Autodesk Fusion 360 part; units mm, degrees
(part 2 of 2)
sketch "スケッチ6" plane through (0, 0, 2) normal (0, 0, 1) x (-1, 0, 0)
  arc A0 (-43.4817, -98.8602) -> (-41.4947, -98.0676) centre (-42.8778, -97.4871) ccw
  arc A1 (41.4947, -98.0676) -> (-41.4947, -98.0676) centre (0, -115.48) ccw
  arc A2 (41.4947, -98.0676) -> (43.4817, -98.8602) centre (42.8778, -97.4871) ccw
  arc A3 (43.4817, -98.8602) -> (50.4167, -95.51) centre (0, 0) ccw
  arc A4 (50.4167, -95.51) -> (51.1376, -90.7356) centre (49.0163, -92.8569) ccw
  line L0 (51.1376, -90.7356) -> (40.8708, -80.4688)
  arc A5 (40.8708, -76.2261) -> (40.8708, -80.4688) centre (42.9921, -78.3474) ccw
  line L1 (40.8708, -76.2261) -> (76.2261, -40.8708)
  arc A6 (80.4688, -40.8708) -> (76.2261, -40.8708) centre (78.3474, -42.9921) ccw
  line L2 (80.4688, -40.8708) -> (90.7356, -51.1376)
  arc A7 (90.7356, -51.1376) -> (95.51, -50.4167) centre (92.8569, -49.0163) ccw
  arc A8 (95.51, -50.4167) -> (95.51, 50.4167) centre (0, 0) ccw
  arc A9 (95.51, 50.4167) -> (90.7356, 51.1376) centre (92.8569, 49.0163) ccw
  line L3 (90.7356, 51.1376) -> (80.4688, 40.8708)
  arc A10 (76.2261, 40.8708) -> (80.4688, 40.8708) centre (78.3474, 42.9921) ccw
  line L4 (76.2261, 40.8708) -> (40.8708, 76.2261)
  arc A11 (40.8708, 80.4688) -> (40.8708, 76.2261) centre (42.9921, 78.3474) ccw
  line L5 (40.8708, 80.4688) -> (51.1376, 90.7356)
  arc A12 (51.1376, 90.7356) -> (50.4167, 95.51) centre (49.0163, 92.8569) ccw
  arc A13 (50.4167, 95.51) -> (-50.4167, 95.51) centre (0, 0) ccw
  arc A14 (-50.4167, 95.51) -> (-51.1376, 90.7356) centre (-49.0163, 92.8569) ccw
  line L6 (-51.1376, 90.7356) -> (-40.8708, 80.4688)
  arc A15 (-40.8708, 76.2261) -> (-40.8708, 80.4688) centre (-42.9921, 78.3474) ccw
  line L7 (-40.8708, 76.2261) -> (-76.2261, 40.8708)
  arc A16 (-80.4688, 40.8708) -> (-76.2261, 40.8708) centre (-78.3474, 42.9921) ccw
  line L8 (-80.4688, 40.8708) -> (-90.7356, 51.1376)
  arc A17 (-90.7356, 51.1376) -> (-95.51, 50.4167) centre (-92.8569, 49.0163) ccw
  arc A18 (-95.51, 50.4167) -> (-95.51, -50.4167) centre (0, 0) ccw
  arc A19 (-95.51, -50.4167) -> (-90.7356, -51.1376) centre (-92.8569, -49.0163) ccw
  line L9 (-90.7356, -51.1376) -> (-80.4688, -40.8708)
  arc A20 (-76.2261, -40.8708) -> (-80.4688, -40.8708) centre (-78.3474, -42.9921) ccw
  line L10 (-76.2261, -40.8708) -> (-40.8708, -76.2261)
  arc A21 (-40.8708, -80.4688) -> (-40.8708, -76.2261) centre (-42.9921, -78.3474) ccw
  line L11 (-40.8708, -80.4688) -> (-51.1376, -90.7356)
  arc A22 (-51.1376, -90.7356) -> (-50.4167, -95.51) centre (-49.0163, -92.8569) ccw
  arc A23 (-50.4167, -95.51) -> (-43.4817, -98.8602) centre (0, 0) ccw
  arc A24 (-38.4462, 71.5797) -> (-36.9817, 75.1152) centre (-41.9817, 75.1152) ccw
  line L12 (-36.9817, 75.1152) -> (-36.9817, 81.5797)
  arc A25 (-36.9817, 81.5797) -> (-38.4462, 85.1152) centre (-41.9817, 81.5797) ccw
  line L13 (-38.4462, 85.1152) -> (-43.658, 90.3271)
  arc A26 (-43.0803, 93.5579) -> (-43.658, 90.3271) centre (-42.2438, 91.7413) ccw
  arc A27 (43.0803, 93.5579) -> (-43.0803, 93.5579) centre (0, 0) ccw
  arc A28 (43.658, 90.3271) -> (43.0803, 93.5579) centre (42.2438, 91.7413) ccw
  line L14 (43.658, 90.3271) -> (38.4462, 85.1152)
  arc A29 (38.4462, 85.1152) -> (36.9817, 81.5797) centre (41.9817, 81.5797) ccw
  line L15 (36.9817, 81.5797) -> (36.9817, 75.1152)
  arc A30 (36.9817, 75.1152) -> (38.4462, 71.5797) centre (41.9817, 75.1152) ccw
  line L16 (38.4462, 71.5797) -> (46.8812, 63.1446)
  arc A31 (46.8812, 58.902) -> (46.8812, 63.1446) centre (44.7599, 61.0233) ccw
  line L17 (46.8812, 58.902) -> (39.0462, 51.0671)
  arc A32 (35.1702, 49.6142) -> (39.0462, 51.0671) centre (35.5107, 54.6026) ccw
  arc A33 (35.1702, 49.6142) -> (32.5058, 46.9498) centre (35, 47.12) ccw
  arc A34 (31.0529, 43.0738) -> (32.5058, 46.9498) centre (27.5174, 46.6093) ccw
  line L18 (31.0529, 43.0738) -> (11.7378, 23.7586)
  arc A35 (11.7378, 23.7586) -> (-9.9511, 24.5606) centre (0, 0) ccw
  arc A36 (-13.199, 25.2198) -> (-9.9511, 24.5606) centre (-11.0776, 27.3411) ccw
  line L19 (-13.199, 25.2198) -> (-31.0529, 43.0738)
  arc A37 (-32.5058, 46.9498) -> (-31.0529, 43.0738) centre (-27.5174, 46.6093) ccw
  arc A38 (-32.5058, 46.9498) -> (-35.1702, 49.6142) centre (-35, 47.12) ccw
  arc A39 (-39.0462, 51.0671) -> (-35.1702, 49.6142) centre (-35.5107, 54.6026) ccw
  line L20 (-39.0462, 51.0671) -> (-46.8812, 58.902)
  arc A40 (-46.8812, 63.1446) -> (-46.8812, 58.902) centre (-44.7599, 61.0233) ccw
  line L21 (-46.8812, 63.1446) -> (-38.4462, 71.5797)
  arc A41 (-72.6906, -37.3352) -> (-84.0043, -37.3352) centre (-78.3474, -42.9921) ccw
  line L22 (-84.0043, -37.3352) -> (-90.3271, -43.658)
  arc A42 (-93.5579, -43.0803) -> (-90.3271, -43.658) centre (-91.7413, -42.2438) ccw
  arc A43 (-93.5579, 43.0803) -> (-93.5579, -43.0803) centre (0, 0) ccw
  arc A44 (-90.3271, 43.658) -> (-93.5579, 43.0803) centre (-91.7413, 42.2438) ccw
  line L23 (-90.3271, 43.658) -> (-84.0043, 37.3352)
  arc A45 (-84.0043, 37.3352) -> (-72.6906, 37.3352) centre (-78.3474, 42.9921) ccw
  line L24 (-72.6906, 37.3352) -> (-63.1446, 46.8812)
  arc A46 (-58.902, 46.8812) -> (-63.1446, 46.8812) centre (-61.0233, 44.7599) ccw
  line L25 (-58.902, 46.8812) -> (-42.5942, 30.5734)
  arc A47 (-42.1845, 26.8416) -> (-42.5942, 30.5734) centre (-44.7155, 28.4521) ccw
  arc A48 (-42.1845, 26.8416) -> (-42.1845, -26.8416) centre (0, 0) ccw
  arc A49 (-42.5942, -30.5734) -> (-42.1845, -26.8416) centre (-44.7155, -28.4521) ccw
  line L26 (-42.5942, -30.5734) -> (-58.902, -46.8812)
  arc A50 (-63.1446, -46.8812) -> (-58.902, -46.8812) centre (-61.0233, -44.7599) ccw
  line L27 (-63.1446, -46.8812) -> (-72.6906, -37.3352)
  arc A51 (72.6906, 37.3352) -> (84.0043, 37.3352) centre (78.3474, 42.9921) ccw
  line L28 (84.0043, 37.3352) -> (90.3271, 43.658)
  arc A52 (93.5579, 43.0803) -> (90.3271, 43.658) centre (91.7413, 42.2438) ccw
  arc A53 (93.5579, -43.0803) -> (93.5579, 43.0803) centre (0, 0) ccw
  arc A54 (90.3271, -43.658) -> (93.5579, -43.0803) centre (91.7413, -42.2438) ccw
  line L29 (90.3271, -43.658) -> (84.0043, -37.3352)
  arc A55 (84.0043, -37.3352) -> (72.6906, -37.3352) centre (78.3474, -42.9921) ccw
  line L30 (72.6906, -37.3352) -> (63.1446, -46.8812)
  arc A56 (58.902, -46.8812) -> (63.1446, -46.8812) centre (61.0233, -44.7599) ccw
  line L31 (58.902, -46.8812) -> (42.5942, -30.5734)
  arc A57 (42.1845, -26.8416) -> (42.5942, -30.5734) centre (44.7155, -28.4521) ccw
  arc A58 (42.1845, -26.8416) -> (42.1845, 26.8416) centre (0, 0) ccw
  arc A59 (42.5942, 30.5734) -> (42.1845, 26.8416) centre (44.7155, 28.4521) ccw
  line L32 (42.5942, 30.5734) -> (58.902, 46.8812)
  arc A60 (63.1446, 46.8812) -> (58.902, 46.8812) centre (61.0233, 44.7599) ccw
  line L33 (63.1446, 46.8812) -> (72.6906, 37.3352)
  line L34 (-22.2194, 14.4412) -> (-56.7807, 49.0025)
  arc A61 (-56.7807, 53.2451) -> (-56.7807, 49.0025) centre (-54.6594, 51.1238) ccw
  line L35 (-56.7807, 53.2451) -> (-53.2451, 56.7807)
  arc A62 (-49.0025, 56.7807) -> (-53.2451, 56.7807) centre (-51.1238, 54.6594) ccw
  line L36 (-49.0025, 56.7807) -> (-14.4412, 22.2194)
  arc A63 (-14.4412, 22.2194) -> (-22.2194, 14.4412) centre (0, 0) ccw
  circle A64 centre (-92.7295, 48.1818) radius 1.65
  circle A65 centre (-92.7295, -48.1818) radius 1.65
  line L37 (-34.5739, 22.5531) -> (-26.135, 14.1142)
  arc A66 (-24.9609, 8.8995) -> (-26.135, 14.1142) centre (-29.6706, 10.5787) ccw
  arc A67 (-24.9609, 8.8995) -> (-24.9609, -8.8995) centre (0, 0) ccw
  arc A68 (-26.135, -14.1142) -> (-24.9609, -8.8995) centre (-29.6706, -10.5787) ccw
  line L38 (-26.135, -14.1142) -> (-34.5739, -22.5531)
  arc A69 (-39.3163, -21.8912) -> (-34.5739, -22.5531) centre (-36.6953, -20.4318) ccw
  arc A70 (-39.3163, 21.8912) -> (-39.3163, -21.8912) centre (0, 0) ccw
  arc A71 (-34.5739, 22.5531) -> (-39.3163, 21.8912) centre (-36.6953, 20.4318) ccw
  line L39 (-56.7807, -49.0025) -> (-22.2194, -14.4412)
  arc A72 (-22.2194, -14.4412) -> (-14.4412, -22.2194) centre (0, 0) ccw
  line L40 (-14.4412, -22.2194) -> (-31.1442, -38.9224)
  arc A73 (-34.8932, -40.3823) -> (-31.1442, -38.9224) centre (-34.6797, -35.3868) ccw
  arc A74 (-34.8932, -40.3823) -> (-37.4977, -42.9868) centre (-35, -42.88) ccw
  arc A75 (-38.9576, -46.7358) -> (-37.4977, -42.9868) centre (-42.4932, -43.2003) ccw
  line L41 (-38.9576, -46.7358) -> (-49.0025, -56.7807)
  arc A76 (-53.2451, -56.7807) -> (-49.0025, -56.7807) centre (-51.1238, -54.6594) ccw
  line L42 (-53.2451, -56.7807) -> (-56.7807, -53.2451)
  arc A77 (-56.7807, -49.0025) -> (-56.7807, -53.2451) centre (-54.6594, -51.1238) ccw
  circle A78 centre (-48.1818, -92.7295) radius 1.65
  circle A79 centre (48.1818, -92.7295) radius 1.65
  arc A80 (23.7586, -11.7378) -> (23.7586, 11.7378) centre (0, 0) ccw
  line L43 (23.7586, 11.7378) -> (34.5739, 22.5531)
  arc A81 (39.3163, 21.8912) -> (34.5739, 22.5531) centre (36.6953, 20.4318) ccw
  arc A82 (39.3163, -21.8912) -> (39.3163, 21.8912) centre (0, 0) ccw
  arc A83 (34.5739, -22.5531) -> (39.3163, -21.8912) centre (36.6953, -20.4318) ccw
  line L44 (34.5739, -22.5531) -> (23.7586, -11.7378)
  circle A84 centre (48.1818, 92.7295) radius 1.65
  circle A85 centre (35, 47.12) radius 1.65
  circle A86 centre (-35, 47.12) radius 1.65
  circle A87 centre (45.7881, -12.6183) radius 1.65
  circle A88 centre (35, -42.88) radius 1.65
  line L45 (22.2194, -14.4412) -> (56.7807, -49.0025)
  arc A89 (56.7807, -53.2451) -> (56.7807, -49.0025) centre (54.6594, -51.1238) ccw
  line L46 (56.7807, -53.2451) -> (53.2451, -56.7807)
  arc A90 (49.0025, -56.7807) -> (53.2451, -56.7807) centre (51.1238, -54.6594) ccw
  line L47 (49.0025, -56.7807) -> (38.9576, -46.7358)
  arc A91 (37.4977, -42.9868) -> (38.9576, -46.7358) centre (42.4932, -43.2003) ccw
  arc A92 (37.4977, -42.9868) -> (34.8932, -40.3823) centre (35, -42.88) ccw
  arc A93 (31.1442, -38.9224) -> (34.8932, -40.3823) centre (34.6797, -35.3868) ccw
  line L48 (31.1442, -38.9224) -> (14.4412, -22.2194)
  arc A94 (14.4412, -22.2194) -> (22.2194, -14.4412) centre (0, 0) ccw
  circle A95 centre (92.7295, -48.1818) radius 1.65
  circle A96 centre (92.7295, 48.1818) radius 1.65
  line L49 (53.2451, 56.7807) -> (56.7807, 53.2451)
  arc A97 (56.7807, 49.0025) -> (56.7807, 53.2451) centre (54.6594, 51.1238) ccw
  line L50 (56.7807, 49.0025) -> (22.2194, 14.4412)
  arc A98 (22.2194, 14.4412) -> (14.4412, 22.2194) centre (0, 0) ccw
  line L51 (14.4412, 22.2194) -> (49.0025, 56.7807)
  arc A99 (53.2451, 56.7807) -> (49.0025, 56.7807) centre (51.1238, 54.6594) ccw
  line L52 (9, -66.2967) -> (9, -24.9249)
  line L53 (11.7378, -23.7586) -> (46.8812, -58.902)
  arc A100 (46.8812, -63.1446) -> (46.8812, -58.902) centre (44.7599, -61.0233) ccw
  line L54 (46.8812, -63.1446) -> (34.4346, -75.5912)
  arc A101 (30.4842, -75.8478) -> (34.4346, -75.5912) centre (32.3133, -73.4699) ccw
  arc A102 (30.4842, -75.8478) -> (9, -66.2967) centre (0, -115.48) ccw
  arc A103 (6, -65.8413) -> (-6, -65.8413) centre (0, -115.48) ccw
  line L55 (-6, -65.8413) -> (-6, -25.8118)
  arc A104 (-6, -25.8118) -> (6, -25.8118) centre (0, 0) ccw
  line L56 (6, -25.8118) -> (6, -65.8413)
  circle A105 centre (-45.7881, -12.6183) radius 1.65
  line L57 (-46.8812, -58.902) -> (-11.7378, -23.7586)
  line L58 (-9, -24.9249) -> (-9, -66.2967)
  arc A106 (-9, -66.2967) -> (-30.4842, -75.8478) centre (0, -115.48) ccw
  arc A107 (-34.4346, -75.5912) -> (-30.4842, -75.8478) centre (-32.3133, -73.4699) ccw
  line L59 (-34.4346, -75.5912) -> (-46.8812, -63.1446)
  arc A108 (-46.8812, -58.902) -> (-46.8812, -63.1446) centre (-44.7599, -61.0233) ccw
  circle A109 centre (-35, -42.88) radius 1.65
  circle A110 centre (0, 0) radius 23.5
  circle A111 centre (-48.1818, 92.7295) radius 1.65
  line L60 (43.2721, 31.2513) -> (33.8603, 21.8395)
  circle A112 centre (0, 0) radius 50
  circle A113 centre (0, 0) radius 45
  line L61 (40.8511, 28.8303) -> (43.8511, 28.8303)
  circle A114 centre (43.8511, 28.8303) radius 2.5
  circle A115 centre (43.8511, 28.8303) radius 1.65
  line L62 (0, -2.5) -> (0, -20)
  circle A116 centre (-43.8511, 28.8303) radius 2.5
  circle A117 centre (-43.8511, 28.8303) radius 1.65
  arc A118 (9, -24.9249) -> (11.7378, -23.7586) centre (0, 0) ccw
  arc A119 (-11.7378, -23.7586) -> (-9, -24.9249) centre (0, 0) ccw
  dimension "d249" = 3
  dimension "d250" = 5
  dimension "d251" = 3.3
  constraint coincident L32 L60.start
  constraint coincident L43 L60.end
  constraint concentric A3 A112
  constraint coincident A3.centre A8.centre
  constraint coincident A112 L61.start
  constraint coincident L60 L61.start
  constraint horizontal L61
  constraint coincident L61.end A114.centre
  constraint concentric A114 A115
  constraint symmetric A114 L62 A116
  constraint symmetric A115 L62 A117
  measures "d249" distance of L61.start L61.end
  measures "d250" diameter of A114
  measures "d251" diameter of A115
extrude "押し出し9" add sketch "スケッチ6" against normal blind 2 contours L25 A47 A116 | A59 L32 L60 A114
fillet "フィレット34" radius 3 2 edges at (-23.7586, 11.7378, 1) (-23.7586, -11.7378, 1)
fillet "フィレット35" radius 4 4 edges at (-42.0273, -27.1204, 1) (-43.2865, -31.2657, 1) (43.2865, -31.2657, 1) (42.0273, -27.1204, 1)
sketch "スケッチ7" plane through (0, 0, 2) normal (0, 0, 1) x (-1, 0, 0)
  circle A0 centre (-43.8511, 28.8303) radius 1.65
  circle A1 centre (43.8511, 28.8303) radius 1.65
  arc A2 (-43.4817, -98.8602) -> (-41.4947, -98.0676) centre (-42.8778, -97.4871) ccw
  arc A3 (41.4947, -98.0676) -> (-41.4947, -98.0676) centre (0, -115.48) ccw
  arc A4 (41.4947, -98.0676) -> (43.4817, -98.8602) centre (42.8778, -97.4871) ccw
  arc A5 (43.4817, -98.8602) -> (50.4167, -95.51) centre (0, 0) ccw
  arc A6 (50.4167, -95.51) -> (51.1376, -90.7356) centre (49.0163, -92.8569) ccw
  line L0 (51.1376, -90.7356) -> (40.8708, -80.4688)
  arc A7 (40.8708, -76.2261) -> (40.8708, -80.4688) centre (42.9921, -78.3474) ccw
  line L1 (40.8708, -76.2261) -> (76.2261, -40.8708)
  arc A8 (80.4688, -40.8708) -> (76.2261, -40.8708) centre (78.3474, -42.9921) ccw
  line L2 (80.4688, -40.8708) -> (90.7356, -51.1376)
  arc A9 (90.7356, -51.1376) -> (95.51, -50.4167) centre (92.8569, -49.0163) ccw
  arc A10 (95.51, -50.4167) -> (95.51, 50.4167) centre (0, 0) ccw
  arc A11 (95.51, 50.4167) -> (90.7356, 51.1376) centre (92.8569, 49.0163) ccw
  line L3 (90.7356, 51.1376) -> (80.4688, 40.8708)
  arc A12 (76.2261, 40.8708) -> (80.4688, 40.8708) centre (78.3474, 42.9921) ccw
  line L4 (76.2261, 40.8708) -> (40.8708, 76.2261)
  arc A13 (40.8708, 80.4688) -> (40.8708, 76.2261) centre (42.9921, 78.3474) ccw
  line L5 (40.8708, 80.4688) -> (51.1376, 90.7356)
  arc A14 (51.1376, 90.7356) -> (50.4167, 95.51) centre (49.0163, 92.8569) ccw
  arc A15 (50.4167, 95.51) -> (-50.4167, 95.51) centre (0, 0) ccw
  arc A16 (-50.4167, 95.51) -> (-51.1376, 90.7356) centre (-49.0163, 92.8569) ccw
  line L6 (-51.1376, 90.7356) -> (-40.8708, 80.4688)
  arc A17 (-40.8708, 76.2261) -> (-40.8708, 80.4688) centre (-42.9921, 78.3474) ccw
  line L7 (-40.8708, 76.2261) -> (-76.2261, 40.8708)
  arc A18 (-80.4688, 40.8708) -> (-76.2261, 40.8708) centre (-78.3474, 42.9921) ccw
  line L8 (-80.4688, 40.8708) -> (-90.7356, 51.1376)
  arc A19 (-90.7356, 51.1376) -> (-95.51, 50.4167) centre (-92.8569, 49.0163) ccw
  arc A20 (-95.51, 50.4167) -> (-95.51, -50.4167) centre (0, 0) ccw
  arc A21 (-95.51, -50.4167) -> (-90.7356, -51.1376) centre (-92.8569, -49.0163) ccw
  line L9 (-90.7356, -51.1376) -> (-80.4688, -40.8708)
  arc A22 (-76.2261, -40.8708) -> (-80.4688, -40.8708) centre (-78.3474, -42.9921) ccw
  line L10 (-76.2261, -40.8708) -> (-40.8708, -76.2261)
  arc A23 (-40.8708, -80.4688) -> (-40.8708, -76.2261) centre (-42.9921, -78.3474) ccw
  line L11 (-40.8708, -80.4688) -> (-51.1376, -90.7356)
  arc A24 (-51.1376, -90.7356) -> (-50.4167, -95.51) centre (-49.0163, -92.8569) ccw
  arc A25 (-50.4167, -95.51) -> (-43.4817, -98.8602) centre (0, 0) ccw
  arc A26 (-38.4462, 71.5797) -> (-36.9817, 75.1152) centre (-41.9817, 75.1152) ccw
  line L12 (-36.9817, 75.1152) -> (-36.9817, 81.5797)
  arc A27 (-36.9817, 81.5797) -> (-38.4462, 85.1152) centre (-41.9817, 81.5797) ccw
  line L13 (-38.4462, 85.1152) -> (-43.658, 90.3271)
  arc A28 (-43.0803, 93.5579) -> (-43.658, 90.3271) centre (-42.2438, 91.7413) ccw
  arc A29 (43.0803, 93.5579) -> (-43.0803, 93.5579) centre (0, 0) ccw
  arc A30 (43.658, 90.3271) -> (43.0803, 93.5579) centre (42.2438, 91.7413) ccw
  line L14 (43.658, 90.3271) -> (38.4462, 85.1152)
  arc A31 (38.4462, 85.1152) -> (36.9817, 81.5797) centre (41.9817, 81.5797) ccw
  line L15 (36.9817, 81.5797) -> (36.9817, 75.1152)
  arc A32 (36.9817, 75.1152) -> (38.4462, 71.5797) centre (41.9817, 75.1152) ccw
  line L16 (38.4462, 71.5797) -> (46.8812, 63.1446)
  arc A33 (46.8812, 58.902) -> (46.8812, 63.1446) centre (44.7599, 61.0233) ccw
  line L17 (46.8812, 58.902) -> (39.0462, 51.0671)
  arc A34 (35.1702, 49.6142) -> (39.0462, 51.0671) centre (35.5107, 54.6026) ccw
  arc A35 (35.1702, 49.6142) -> (32.5058, 46.9498) centre (35, 47.12) ccw
  arc A36 (31.0529, 43.0738) -> (32.5058, 46.9498) centre (27.5174, 46.6093) ccw
  line L18 (31.0529, 43.0738) -> (11.7378, 23.7586)
  arc A37 (11.7378, 23.7586) -> (-9.9511, 24.5606) centre (0, 0) ccw
  arc A38 (-13.199, 25.2198) -> (-9.9511, 24.5606) centre (-11.0776, 27.3411) ccw
  line L19 (-13.199, 25.2198) -> (-31.0529, 43.0738)
  arc A39 (-32.5058, 46.9498) -> (-31.0529, 43.0738) centre (-27.5174, 46.6093) ccw
  arc A40 (-32.5058, 46.9498) -> (-35.1702, 49.6142) centre (-35, 47.12) ccw
  arc A41 (-39.0462, 51.0671) -> (-35.1702, 49.6142) centre (-35.5107, 54.6026) ccw
  line L20 (-39.0462, 51.0671) -> (-46.8812, 58.902)
  arc A42 (-46.8812, 63.1446) -> (-46.8812, 58.902) centre (-44.7599, 61.0233) ccw
  line L21 (-46.8812, 63.1446) -> (-38.4462, 71.5797)
  arc A43 (-72.6906, -37.3352) -> (-84.0043, -37.3352) centre (-78.3474, -42.9921) ccw
  line L22 (-84.0043, -37.3352) -> (-90.3271, -43.658)
  arc A44 (-93.5579, -43.0803) -> (-90.3271, -43.658) centre (-91.7413, -42.2438) ccw
  arc A45 (-93.5579, 43.0803) -> (-93.5579, -43.0803) centre (0, 0) ccw
  arc A46 (-90.3271, 43.658) -> (-93.5579, 43.0803) centre (-91.7413, 42.2438) ccw
  line L23 (-90.3271, 43.658) -> (-84.0043, 37.3352)
  arc A47 (-84.0043, 37.3352) -> (-72.6906, 37.3352) centre (-78.3474, 42.9921) ccw
  line L24 (-72.6906, 37.3352) -> (-63.1446, 46.8812)
  arc A48 (-58.902, 46.8812) -> (-63.1446, 46.8812) centre (-61.0233, 44.7599) ccw
  line L25 (-58.902, 46.8812) -> (-46.7511, 34.7303)
  arc A49 (-46.0544, 30.0117) -> (-46.7511, 34.7303) centre (-49.5796, 31.9019) ccw
  arc A50 (-46.0544, 30.0117) -> (-45.5696, 27.0146) centre (-43.8511, 28.8303) ccw
  arc A51 (-44.7399, 22.3235) -> (-45.5696, 27.0146) centre (-48.3191, 24.1094) ccw
  arc A52 (-44.7399, 22.3235) -> (-42.1845, -26.8416) centre (0, 0) ccw
  arc A53 (-42.5942, -30.5734) -> (-42.1845, -26.8416) centre (-44.7155, -28.4521) ccw
  line L26 (-42.5942, -30.5734) -> (-58.902, -46.8812)
  arc A54 (-63.1446, -46.8812) -> (-58.902, -46.8812) centre (-61.0233, -44.7599) ccw
  line L27 (-63.1446, -46.8812) -> (-72.6906, -37.3352)
  arc A55 (72.6906, 37.3352) -> (84.0043, 37.3352) centre (78.3474, 42.9921) ccw
  line L28 (84.0043, 37.3352) -> (90.3271, 43.658)
  arc A56 (93.5579, 43.0803) -> (90.3271, 43.658) centre (91.7413, 42.2438) ccw
  arc A57 (93.5579, -43.0803) -> (93.5579, 43.0803) centre (0, 0) ccw
  arc A58 (90.3271, -43.658) -> (93.5579, -43.0803) centre (91.7413, -42.2438) ccw
  line L29 (90.3271, -43.658) -> (84.0043, -37.3352)
  arc A59 (84.0043, -37.3352) -> (72.6906, -37.3352) centre (78.3474, -42.9921) ccw
  line L30 (72.6906, -37.3352) -> (63.1446, -46.8812)
  arc A60 (58.902, -46.8812) -> (63.1446, -46.8812) centre (61.0233, -44.7599) ccw
  line L31 (58.902, -46.8812) -> (42.5942, -30.5734)
  arc A61 (42.1845, -26.8416) -> (42.5942, -30.5734) centre (44.7155, -28.4521) ccw
  arc A62 (42.1845, -26.8416) -> (44.7399, 22.3235) centre (0, 0) ccw
  arc A63 (45.5696, 27.0146) -> (44.7399, 22.3235) centre (48.3191, 24.1094) ccw
  arc A64 (45.5696, 27.0146) -> (46.0544, 30.0117) centre (43.8511, 28.8303) ccw
  arc A65 (46.7511, 34.7303) -> (46.0544, 30.0117) centre (49.5796, 31.9019) ccw
  line L32 (46.7511, 34.7303) -> (58.902, 46.8812)
  arc A66 (63.1446, 46.8812) -> (58.902, 46.8812) centre (61.0233, 44.7599) ccw
  line L33 (63.1446, 46.8812) -> (72.6906, 37.3352)
  line L34 (-22.2194, 14.4412) -> (-56.7807, 49.0025)
  arc A67 (-56.7807, 53.2451) -> (-56.7807, 49.0025) centre (-54.6594, 51.1238) ccw
  line L35 (-56.7807, 53.2451) -> (-53.2451, 56.7807)
  arc A68 (-49.0025, 56.7807) -> (-53.2451, 56.7807) centre (-51.1238, 54.6594) ccw
  line L36 (-49.0025, 56.7807) -> (-14.4412, 22.2194)
  arc A69 (-14.4412, 22.2194) -> (-22.2194, 14.4412) centre (0, 0) ccw
  circle A70 centre (-92.7295, 48.1818) radius 1.65
  circle A71 centre (-92.7295, -48.1818) radius 1.65
  line L37 (-34.5739, 22.5531) -> (-26.135, 14.1142)
  arc A72 (-24.9609, 8.8995) -> (-26.135, 14.1142) centre (-29.6706, 10.5787) ccw
  arc A73 (-24.9609, 8.8995) -> (-24.9609, -8.8995) centre (0, 0) ccw
  arc A74 (-26.135, -14.1142) -> (-24.9609, -8.8995) centre (-29.6706, -10.5787) ccw
  line L38 (-26.135, -14.1142) -> (-34.5739, -22.5531)
  arc A75 (-39.3163, -21.8912) -> (-34.5739, -22.5531) centre (-36.6953, -20.4318) ccw
  arc A76 (-39.3163, 21.8912) -> (-39.3163, -21.8912) centre (0, 0) ccw
  arc A77 (-34.5739, 22.5531) -> (-39.3163, 21.8912) centre (-36.6953, 20.4318) ccw
  line L39 (-56.7807, -49.0025) -> (-22.2194, -14.4412)
  arc A78 (-22.2194, -14.4412) -> (-14.4412, -22.2194) centre (0, 0) ccw
  line L40 (-14.4412, -22.2194) -> (-31.1442, -38.9224)
  arc A79 (-34.8932, -40.3823) -> (-31.1442, -38.9224) centre (-34.6797, -35.3868) ccw
  arc A80 (-34.8932, -40.3823) -> (-37.4977, -42.9868) centre (-35, -42.88) ccw
  arc A81 (-38.9576, -46.7358) -> (-37.4977, -42.9868) centre (-42.4932, -43.2003) ccw
  line L41 (-38.9576, -46.7358) -> (-49.0025, -56.7807)
  arc A82 (-53.2451, -56.7807) -> (-49.0025, -56.7807) centre (-51.1238, -54.6594) ccw
  line L42 (-53.2451, -56.7807) -> (-56.7807, -53.2451)
  arc A83 (-56.7807, -49.0025) -> (-56.7807, -53.2451) centre (-54.6594, -51.1238) ccw
  circle A84 centre (-48.1818, -92.7295) radius 1.65
  circle A85 centre (48.1818, -92.7295) radius 1.65
  arc A86 (24.5606, -9.9511) -> (24.5606, 9.9511) centre (0, 0) ccw
  arc A87 (25.2198, 13.199) -> (24.5606, 9.9511) centre (27.3411, 11.0776) ccw
  line L43 (25.2198, 13.199) -> (34.5739, 22.5531)
  arc A88 (39.3163, 21.8912) -> (34.5739, 22.5531) centre (36.6953, 20.4318) ccw
  arc A89 (39.3163, -21.8912) -> (39.3163, 21.8912) centre (0, 0) ccw
  arc A90 (34.5739, -22.5531) -> (39.3163, -21.8912) centre (36.6953, -20.4318) ccw
  line L44 (34.5739, -22.5531) -> (25.2198, -13.199)
  arc A91 (24.5606, -9.9511) -> (25.2198, -13.199) centre (27.3411, -11.0776) ccw
  circle A92 centre (48.1818, 92.7295) radius 1.65
  circle A93 centre (35, 47.12) radius 1.65
  circle A94 centre (-35, 47.12) radius 1.65
  circle A95 centre (45.7881, -12.6183) radius 1.65
  circle A96 centre (35, -42.88) radius 1.65
  line L45 (22.2194, -14.4412) -> (56.7807, -49.0025)
  arc A97 (56.7807, -53.2451) -> (56.7807, -49.0025) centre (54.6594, -51.1238) ccw
  line L46 (56.7807, -53.2451) -> (53.2451, -56.7807)
  arc A98 (49.0025, -56.7807) -> (53.2451, -56.7807) centre (51.1238, -54.6594) ccw
  line L47 (49.0025, -56.7807) -> (38.9576, -46.7358)
  arc A99 (37.4977, -42.9868) -> (38.9576, -46.7358) centre (42.4932, -43.2003) ccw
  arc A100 (37.4977, -42.9868) -> (34.8932, -40.3823) centre (35, -42.88) ccw
  arc A101 (31.1442, -38.9224) -> (34.8932, -40.3823) centre (34.6797, -35.3868) ccw
  line L48 (31.1442, -38.9224) -> (14.4412, -22.2194)
  arc A102 (14.4412, -22.2194) -> (22.2194, -14.4412) centre (0, 0) ccw
  circle A103 centre (92.7295, -48.1818) radius 1.65
  circle A104 centre (92.7295, 48.1818) radius 1.65
  line L49 (53.2451, 56.7807) -> (56.7807, 53.2451)
  arc A105 (56.7807, 49.0025) -> (56.7807, 53.2451) centre (54.6594, 51.1238) ccw
  line L50 (56.7807, 49.0025) -> (22.2194, 14.4412)
  arc A106 (22.2194, 14.4412) -> (14.4412, 22.2194) centre (0, 0) ccw
  line L51 (14.4412, 22.2194) -> (49.0025, 56.7807)
  arc A107 (53.2451, 56.7807) -> (49.0025, 56.7807) centre (51.1238, 54.6594) ccw
  line L52 (9, -66.2967) -> (9, -24.9249)
  arc A108 (9, -24.9249) -> (11.7378, -23.7586) centre (0, 0) ccw
  line L53 (11.7378, -23.7586) -> (46.8812, -58.902)
  arc A109 (46.8812, -63.1446) -> (46.8812, -58.902) centre (44.7599, -61.0233) ccw
  line L54 (46.8812, -63.1446) -> (34.4346, -75.5912)
  arc A110 (30.4842, -75.8478) -> (34.4346, -75.5912) centre (32.3133, -73.4699) ccw
  arc A111 (30.4842, -75.8478) -> (9, -66.2967) centre (0, -115.48) ccw
  arc A112 (6, -65.8413) -> (-6, -65.8413) centre (0, -115.48) ccw
  line L55 (-6, -65.8413) -> (-6, -25.8118)
  arc A113 (-6, -25.8118) -> (6, -25.8118) centre (0, 0) ccw
  line L56 (6, -25.8118) -> (6, -65.8413)
  circle A114 centre (-45.7881, -12.6183) radius 1.65
  line L57 (-46.8812, -58.902) -> (-11.7378, -23.7586)
  arc A115 (-11.7378, -23.7586) -> (-9, -24.9249) centre (0, 0) ccw
  line L58 (-9, -24.9249) -> (-9, -66.2967)
  arc A116 (-9, -66.2967) -> (-30.4842, -75.8478) centre (0, -115.48) ccw
  arc A117 (-34.4346, -75.5912) -> (-30.4842, -75.8478) centre (-32.3133, -73.4699) ccw
  line L59 (-34.4346, -75.5912) -> (-46.8812, -63.1446)
  arc A118 (-46.8812, -58.902) -> (-46.8812, -63.1446) centre (-44.7599, -61.0233) ccw
  circle A119 centre (-35, -42.88) radius 1.65
  circle A120 centre (0, 0) radius 23.5
  circle A121 centre (-48.1818, 92.7295) radius 1.65
  line L60 (0, -65.48) -> (13.1, -65.48)
  line L61 (13.1, -65.48) -> (13.1, -25.1208)
  line L62 (13.1, -25.1208) -> (16.1, -25.1208)
  line L63 (16.1, -25.1208) -> (16.1, -68.143)
  line L64 (13.1, -65.48) -> (13.1, -67.2266)
  line L65 (0, -65.48) -> (-13.1, -65.48)
  line L66 (-13.1, -65.48) -> (-13.1, -25.1208)
  line L67 (-13.1, -65.48) -> (-16.1, -65.48)
  line L68 (-16.1, -65.48) -> (-16.1, -68.143)
  line L69 (-13.1, -65.48) -> (-13.1, -67.2266)
  line L70 (-16.1, -65.48) -> (-16.1, -28.1208)
  dimension "d258" = 13.1
  dimension "d259" = 3
  dimension "d260" = 13.1
  dimension "d261" = 3
  constraint midpoint A112 L60.start
  constraint perpendicular L56 L60
  constraint coincident L53 L61.end
  constraint perpendicular L60 L61
  constraint perpendicular L61 L62
  constraint coincident A111 L63.end
  constraint perpendicular L62 L63
  constraint coincident A111 L64.end
  constraint perpendicular L60 L64
  constraint perpendicular L58 L65
  constraint coincident L57 L66.end
  constraint perpendicular L65 L66
  constraint perpendicular L66 L67
  constraint coincident A116 L68.end
  constraint perpendicular L65 L68
  constraint coincident A116 L69.end
  constraint perpendicular L67 L69
  constraint coincident L57 L70.end
  constraint perpendicular L67 L70
  measures "d258" distance of L60.start L60.end
  measures "d259" distance of L61.end L62.end
  measures "d260" distance of L60.start L65.end
  measures "d261" distance of L65.end L67.end
extrude "押し出し10" add sketch "スケッチ7" against normal blind 2 contours L53 A111 L61 L63 L64 | L57 L66 L67 L70 | A116 L67 L68 L69
sketch "スケッチ8" plane through (0, 0, 2) normal (0, 0, 1) x (-1, 0, 0)
  line L0 (-13.1, -25.1208) -> (-11.7378, -23.7586)
  arc A0 (-11.7378, -23.7586) -> (-9, -24.9249) centre (0, 0) ccw
  line L1 (-9, -24.9249) -> (-9, -66.2967)
  arc A1 (-9, -66.2967) -> (-13.1, -67.2266) centre (0, -115.48) ccw
  line L2 (-13.1, -67.2266) -> (-13.1, -25.1208)
  arc A2 (13.1, -67.2266) -> (9, -66.2967) centre (0, -115.48) ccw
  line L3 (9, -66.2967) -> (9, -24.9249)
  arc A3 (9, -24.9249) -> (11.7378, -23.7586) centre (0, 0) ccw
  line L4 (11.7378, -23.7586) -> (13.1, -25.1208)
  line L5 (13.1, -25.1208) -> (13.1, -67.2266)
  circle A4 centre (-43.8511, 28.8303) radius 1.65
  circle A5 centre (43.8511, 28.8303) radius 1.65
  arc A6 (-43.4817, -98.8602) -> (-41.4947, -98.0676) centre (-42.8778, -97.4871) ccw
  arc A7 (41.4947, -98.0676) -> (-41.4947, -98.0676) centre (0, -115.48) ccw
  arc A8 (41.4947, -98.0676) -> (43.4817, -98.8602) centre (42.8778, -97.4871) ccw
  arc A9 (43.4817, -98.8602) -> (50.4167, -95.51) centre (0, 0) ccw
  arc A10 (50.4167, -95.51) -> (51.1376, -90.7356) centre (49.0163, -92.8569) ccw
  line L6 (51.1376, -90.7356) -> (40.8708, -80.4688)
  arc A11 (40.8708, -76.2261) -> (40.8708, -80.4688) centre (42.9921, -78.3474) ccw
  line L7 (40.8708, -76.2261) -> (76.2261, -40.8708)
  arc A12 (80.4688, -40.8708) -> (76.2261, -40.8708) centre (78.3474, -42.9921) ccw
  line L8 (80.4688, -40.8708) -> (90.7356, -51.1376)
  arc A13 (90.7356, -51.1376) -> (95.51, -50.4167) centre (92.8569, -49.0163) ccw
  arc A14 (95.51, -50.4167) -> (95.51, 50.4167) centre (0, 0) ccw
  arc A15 (95.51, 50.4167) -> (90.7356, 51.1376) centre (92.8569, 49.0163) ccw
  line L9 (90.7356, 51.1376) -> (80.4688, 40.8708)
  arc A16 (76.2261, 40.8708) -> (80.4688, 40.8708) centre (78.3474, 42.9921) ccw
  line L10 (76.2261, 40.8708) -> (40.8708, 76.2261)
  arc A17 (40.8708, 80.4688) -> (40.8708, 76.2261) centre (42.9921, 78.3474) ccw
  line L11 (40.8708, 80.4688) -> (51.1376, 90.7356)
  arc A18 (51.1376, 90.7356) -> (50.4167, 95.51) centre (49.0163, 92.8569) ccw
  arc A19 (50.4167, 95.51) -> (-50.4167, 95.51) centre (0, 0) ccw
  arc A20 (-50.4167, 95.51) -> (-51.1376, 90.7356) centre (-49.0163, 92.8569) ccw
  line L12 (-51.1376, 90.7356) -> (-40.8708, 80.4688)
  arc A21 (-40.8708, 76.2261) -> (-40.8708, 80.4688) centre (-42.9921, 78.3474) ccw
  line L13 (-40.8708, 76.2261) -> (-76.2261, 40.8708)
  arc A22 (-80.4688, 40.8708) -> (-76.2261, 40.8708) centre (-78.3474, 42.9921) ccw
  line L14 (-80.4688, 40.8708) -> (-90.7356, 51.1376)
  arc A23 (-90.7356, 51.1376) -> (-95.51, 50.4167) centre (-92.8569, 49.0163) ccw
  arc A24 (-95.51, 50.4167) -> (-95.51, -50.4167) centre (0, 0) ccw
  arc A25 (-95.51, -50.4167) -> (-90.7356, -51.1376) centre (-92.8569, -49.0163) ccw
  line L15 (-90.7356, -51.1376) -> (-80.4688, -40.8708)
  arc A26 (-76.2261, -40.8708) -> (-80.4688, -40.8708) centre (-78.3474, -42.9921) ccw
  line L16 (-76.2261, -40.8708) -> (-40.8708, -76.2261)
  arc A27 (-40.8708, -80.4688) -> (-40.8708, -76.2261) centre (-42.9921, -78.3474) ccw
  line L17 (-40.8708, -80.4688) -> (-51.1376, -90.7356)
  arc A28 (-51.1376, -90.7356) -> (-50.4167, -95.51) centre (-49.0163, -92.8569) ccw
  arc A29 (-50.4167, -95.51) -> (-43.4817, -98.8602) centre (0, 0) ccw
  arc A30 (-38.4462, 71.5797) -> (-36.9817, 75.1152) centre (-41.9817, 75.1152) ccw
  line L18 (-36.9817, 75.1152) -> (-36.9817, 81.5797)
  arc A31 (-36.9817, 81.5797) -> (-38.4462, 85.1152) centre (-41.9817, 81.5797) ccw
  line L19 (-38.4462, 85.1152) -> (-43.658, 90.3271)
  arc A32 (-43.0803, 93.5579) -> (-43.658, 90.3271) centre (-42.2438, 91.7413) ccw
  arc A33 (43.0803, 93.5579) -> (-43.0803, 93.5579) centre (0, 0) ccw
  arc A34 (43.658, 90.3271) -> (43.0803, 93.5579) centre (42.2438, 91.7413) ccw
  line L20 (43.658, 90.3271) -> (38.4462, 85.1152)
  arc A35 (38.4462, 85.1152) -> (36.9817, 81.5797) centre (41.9817, 81.5797) ccw
  line L21 (36.9817, 81.5797) -> (36.9817, 75.1152)
  arc A36 (36.9817, 75.1152) -> (38.4462, 71.5797) centre (41.9817, 75.1152) ccw
  line L22 (38.4462, 71.5797) -> (46.8812, 63.1446)
  arc A37 (46.8812, 58.902) -> (46.8812, 63.1446) centre (44.7599, 61.0233) ccw
  line L23 (46.8812, 58.902) -> (39.0462, 51.0671)
  arc A38 (35.1702, 49.6142) -> (39.0462, 51.0671) centre (35.5107, 54.6026) ccw
  arc A39 (35.1702, 49.6142) -> (32.5058, 46.9498) centre (35, 47.12) ccw
  arc A40 (31.0529, 43.0738) -> (32.5058, 46.9498) centre (27.5174, 46.6093) ccw
  line L24 (31.0529, 43.0738) -> (11.7378, 23.7586)
  arc A41 (11.7378, 23.7586) -> (-9.9511, 24.5606) centre (0, 0) ccw
  arc A42 (-13.199, 25.2198) -> (-9.9511, 24.5606) centre (-11.0776, 27.3411) ccw
  line L25 (-13.199, 25.2198) -> (-31.0529, 43.0738)
  arc A43 (-32.5058, 46.9498) -> (-31.0529, 43.0738) centre (-27.5174, 46.6093) ccw
  arc A44 (-32.5058, 46.9498) -> (-35.1702, 49.6142) centre (-35, 47.12) ccw
  arc A45 (-39.0462, 51.0671) -> (-35.1702, 49.6142) centre (-35.5107, 54.6026) ccw
  line L26 (-39.0462, 51.0671) -> (-46.8812, 58.902)
  arc A46 (-46.8812, 63.1446) -> (-46.8812, 58.902) centre (-44.7599, 61.0233) ccw
  line L27 (-46.8812, 63.1446) -> (-38.4462, 71.5797)
  arc A47 (-72.6906, -37.3352) -> (-84.0043, -37.3352) centre (-78.3474, -42.9921) ccw
  line L28 (-84.0043, -37.3352) -> (-90.3271, -43.658)
  arc A48 (-93.5579, -43.0803) -> (-90.3271, -43.658) centre (-91.7413, -42.2438) ccw
  arc A49 (-93.5579, 43.0803) -> (-93.5579, -43.0803) centre (0, 0) ccw
  arc A50 (-90.3271, 43.658) -> (-93.5579, 43.0803) centre (-91.7413, 42.2438) ccw
  line L29 (-90.3271, 43.658) -> (-84.0043, 37.3352)
  arc A51 (-84.0043, 37.3352) -> (-72.6906, 37.3352) centre (-78.3474, 42.9921) ccw
  line L30 (-72.6906, 37.3352) -> (-63.1446, 46.8812)
  arc A52 (-58.902, 46.8812) -> (-63.1446, 46.8812) centre (-61.0233, 44.7599) ccw
  line L31 (-58.902, 46.8812) -> (-46.7511, 34.7303)
  arc A53 (-46.0544, 30.0117) -> (-46.7511, 34.7303) centre (-49.5796, 31.9019) ccw
  arc A54 (-46.0544, 30.0117) -> (-45.5696, 27.0146) centre (-43.8511, 28.8303) ccw
  arc A55 (-44.7399, 22.3235) -> (-45.5696, 27.0146) centre (-48.3191, 24.1094) ccw
  arc A56 (-44.7399, 22.3235) -> (-42.1845, -26.8416) centre (0, 0) ccw
  arc A57 (-42.5942, -30.5734) -> (-42.1845, -26.8416) centre (-44.7155, -28.4521) ccw
  line L32 (-42.5942, -30.5734) -> (-58.902, -46.8812)
  arc A58 (-63.1446, -46.8812) -> (-58.902, -46.8812) centre (-61.0233, -44.7599) ccw
  line L33 (-63.1446, -46.8812) -> (-72.6906, -37.3352)
  arc A59 (72.6906, 37.3352) -> (84.0043, 37.3352) centre (78.3474, 42.9921) ccw
  line L34 (84.0043, 37.3352) -> (90.3271, 43.658)
  arc A60 (93.5579, 43.0803) -> (90.3271, 43.658) centre (91.7413, 42.2438) ccw
  arc A61 (93.5579, -43.0803) -> (93.5579, 43.0803) centre (0, 0) ccw
  arc A62 (90.3271, -43.658) -> (93.5579, -43.0803) centre (91.7413, -42.2438) ccw
  line L35 (90.3271, -43.658) -> (84.0043, -37.3352)
  arc A63 (84.0043, -37.3352) -> (72.6906, -37.3352) centre (78.3474, -42.9921) ccw
  line L36 (72.6906, -37.3352) -> (63.1446, -46.8812)
  arc A64 (58.902, -46.8812) -> (63.1446, -46.8812) centre (61.0233, -44.7599) ccw
  line L37 (58.902, -46.8812) -> (42.5942, -30.5734)
  arc A65 (42.1845, -26.8416) -> (42.5942, -30.5734) centre (44.7155, -28.4521) ccw
  arc A66 (42.1845, -26.8416) -> (44.7399, 22.3235) centre (0, 0) ccw
  arc A67 (45.5696, 27.0146) -> (44.7399, 22.3235) centre (48.3191, 24.1094) ccw
  arc A68 (45.5696, 27.0146) -> (46.0544, 30.0117) centre (43.8511, 28.8303) ccw
  arc A69 (46.7511, 34.7303) -> (46.0544, 30.0117) centre (49.5796, 31.9019) ccw
  line L38 (46.7511, 34.7303) -> (58.902, 46.8812)
  arc A70 (63.1446, 46.8812) -> (58.902, 46.8812) centre (61.0233, 44.7599) ccw
  line L39 (63.1446, 46.8812) -> (72.6906, 37.3352)
  line L40 (-22.2194, 14.4412) -> (-56.7807, 49.0025)
  arc A71 (-56.7807, 53.2451) -> (-56.7807, 49.0025) centre (-54.6594, 51.1238) ccw
  line L41 (-56.7807, 53.2451) -> (-53.2451, 56.7807)
  arc A72 (-49.0025, 56.7807) -> (-53.2451, 56.7807) centre (-51.1238, 54.6594) ccw
  line L42 (-49.0025, 56.7807) -> (-14.4412, 22.2194)
  arc A73 (-14.4412, 22.2194) -> (-22.2194, 14.4412) centre (0, 0) ccw
  circle A74 centre (-92.7295, 48.1818) radius 1.65
  circle A75 centre (-92.7295, -48.1818) radius 1.65
  line L43 (-34.5739, 22.5531) -> (-26.135, 14.1142)
  arc A76 (-24.9609, 8.8995) -> (-26.135, 14.1142) centre (-29.6706, 10.5787) ccw
  arc A77 (-24.9609, 8.8995) -> (-24.9609, -8.8995) centre (0, 0) ccw
  arc A78 (-26.135, -14.1142) -> (-24.9609, -8.8995) centre (-29.6706, -10.5787) ccw
  line L44 (-26.135, -14.1142) -> (-34.5739, -22.5531)
  arc A79 (-39.3163, -21.8912) -> (-34.5739, -22.5531) centre (-36.6953, -20.4318) ccw
  arc A80 (-39.3163, 21.8912) -> (-39.3163, -21.8912) centre (0, 0) ccw
  arc A81 (-34.5739, 22.5531) -> (-39.3163, 21.8912) centre (-36.6953, 20.4318) ccw
  line L45 (-56.7807, -49.0025) -> (-22.2194, -14.4412)
  arc A82 (-22.2194, -14.4412) -> (-14.4412, -22.2194) centre (0, 0) ccw
  line L46 (-14.4412, -22.2194) -> (-31.1442, -38.9224)
  arc A83 (-34.8932, -40.3823) -> (-31.1442, -38.9224) centre (-34.6797, -35.3868) ccw
  arc A84 (-34.8932, -40.3823) -> (-37.4977, -42.9868) centre (-35, -42.88) ccw
  arc A85 (-38.9576, -46.7358) -> (-37.4977, -42.9868) centre (-42.4932, -43.2003) ccw
  line L47 (-38.9576, -46.7358) -> (-49.0025, -56.7807)
  arc A86 (-53.2451, -56.7807) -> (-49.0025, -56.7807) centre (-51.1238, -54.6594) ccw
  line L48 (-53.2451, -56.7807) -> (-56.7807, -53.2451)
  arc A87 (-56.7807, -49.0025) -> (-56.7807, -53.2451) centre (-54.6594, -51.1238) ccw
  circle A88 centre (-48.1818, -92.7295) radius 1.65
  circle A89 centre (48.1818, -92.7295) radius 1.65
  arc A90 (24.5606, -9.9511) -> (24.5606, 9.9511) centre (0, 0) ccw
  arc A91 (25.2198, 13.199) -> (24.5606, 9.9511) centre (27.3411, 11.0776) ccw
  line L49 (25.2198, 13.199) -> (34.5739, 22.5531)
  arc A92 (39.3163, 21.8912) -> (34.5739, 22.5531) centre (36.6953, 20.4318) ccw
  arc A93 (39.3163, -21.8912) -> (39.3163, 21.8912) centre (0, 0) ccw
  arc A94 (34.5739, -22.5531) -> (39.3163, -21.8912) centre (36.6953, -20.4318) ccw
  line L50 (34.5739, -22.5531) -> (25.2198, -13.199)
  arc A95 (24.5606, -9.9511) -> (25.2198, -13.199) centre (27.3411, -11.0776) ccw
  circle A96 centre (48.1818, 92.7295) radius 1.65
  circle A97 centre (35, 47.12) radius 1.65
  circle A98 centre (-35, 47.12) radius 1.65
  circle A99 centre (45.7881, -12.6183) radius 1.65
  circle A100 centre (35, -42.88) radius 1.65
  line L51 (22.2194, -14.4412) -> (56.7807, -49.0025)
  arc A101 (56.7807, -53.2451) -> (56.7807, -49.0025) centre (54.6594, -51.1238) ccw
  line L52 (56.7807, -53.2451) -> (53.2451, -56.7807)
  arc A102 (49.0025, -56.7807) -> (53.2451, -56.7807) centre (51.1238, -54.6594) ccw
  line L53 (49.0025, -56.7807) -> (38.9576, -46.7358)
  arc A103 (37.4977, -42.9868) -> (38.9576, -46.7358) centre (42.4932, -43.2003) ccw
  arc A104 (37.4977, -42.9868) -> (34.8932, -40.3823) centre (35, -42.88) ccw
  arc A105 (31.1442, -38.9224) -> (34.8932, -40.3823) centre (34.6797, -35.3868) ccw
  line L54 (31.1442, -38.9224) -> (14.4412, -22.2194)
  arc A106 (14.4412, -22.2194) -> (22.2194, -14.4412) centre (0, 0) ccw
  circle A107 centre (92.7295, -48.1818) radius 1.65
  circle A108 centre (92.7295, 48.1818) radius 1.65
  line L55 (53.2451, 56.7807) -> (56.7807, 53.2451)
  arc A109 (56.7807, 49.0025) -> (56.7807, 53.2451) centre (54.6594, 51.1238) ccw
  line L56 (56.7807, 49.0025) -> (22.2194, 14.4412)
  arc A110 (22.2194, 14.4412) -> (14.4412, 22.2194) centre (0, 0) ccw
  line L57 (14.4412, 22.2194) -> (49.0025, 56.7807)
  arc A111 (53.2451, 56.7807) -> (49.0025, 56.7807) centre (51.1238, 54.6594) ccw
  line L58 (16.1, -68.143) -> (16.1, -28.1208)
  line L59 (16.1, -28.1208) -> (46.8812, -58.902)
  arc A112 (46.8812, -63.1446) -> (46.8812, -58.902) centre (44.7599, -61.0233) ccw
  line L60 (46.8812, -63.1446) -> (34.4346, -75.5912)
  arc A113 (30.4842, -75.8478) -> (34.4346, -75.5912) centre (32.3133, -73.4699) ccw
  arc A114 (30.4842, -75.8478) -> (16.1, -68.143) centre (0, -115.48) ccw
  arc A115 (6, -65.8413) -> (-6, -65.8413) centre (0, -115.48) ccw
  line L61 (-6, -65.8413) -> (-6, -25.8118)
  arc A116 (-6, -25.8118) -> (6, -25.8118) centre (0, 0) ccw
  line L62 (6, -25.8118) -> (6, -65.8413)
  circle A117 centre (-45.7881, -12.6183) radius 1.65
  line L63 (-16.1, -28.1208) -> (-16.1, -68.143)
  arc A118 (-16.1, -68.143) -> (-30.4842, -75.8478) centre (0, -115.48) ccw
  arc A119 (-34.4346, -75.5912) -> (-30.4842, -75.8478) centre (-32.3133, -73.4699) ccw
  line L64 (-34.4346, -75.5912) -> (-46.8812, -63.1446)
  arc A120 (-46.8812, -58.902) -> (-46.8812, -63.1446) centre (-44.7599, -61.0233) ccw
  line L65 (-46.8812, -58.902) -> (-16.1, -28.1208)
  circle A121 centre (-35, -42.88) radius 1.65
  circle A122 centre (0, 0) radius 23.5
  circle A123 centre (-48.1818, 92.7295) radius 1.65
  circle A124 centre (0, -115.48) radius 50
  circle A125 centre (0, 0) radius 26.5
  constraint concentric A1 A124
  constraint concentric A0 A125
extrude "押し出し11" cut sketch "スケッチ8" against normal blind 2 contours L1 L61 A124 A125 | L3 L62 A124 A125
fillet "フィレット36" radius 2 9 edges at (-11.7378, 23.7586, 1) (-13.1, 25.1208, 1) (-16.1, 28.1208, 1) (13.1, 25.1208, 1) (16.1, 28.1208, 1) (13.1, 67.2266, 1) (16.1, 68.143, 1) (-16.1, 68.143, 1) (-13.1, 67.2266, 1)
fillet "フィレット37" radius 2 1 edges at (11.7378, 23.7586, 1)
fillet "フィレット38" radius 2 8 edges at (-22.2194, 14.4412, 1) (-14.4412, 22.2194, 1) (-22.2194, -14.4412, 1) (-14.4412, -22.2194, 1) (14.4412, -22.2194, 1) (22.2194, -14.4412, 1) (22.2194, 14.4412, 1) (14.4412, 22.2194, 1)
fillet "フィレット39" radius 3 1 edges at (-11.7378, -23.7586, 1)
